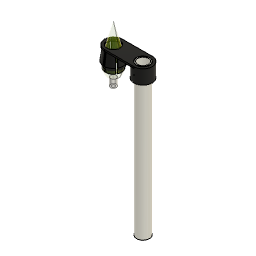
model (Autodesk Fusion 360 design; units mm, degrees)
Autodesk Fusion 360 part; units mm, degrees
note: some values were not read from the file. Chosen so that the rebuilt part matches the saved one: how an offset face is resized. Set by a fixed rule: which sketch regions a step uses.
sketch "Sketch1" plane through (0, 0, 0) normal (0, 0, 1) x (1, 0, 0)
  circle A0 centre (60, 0) radius 13.435
  circle A1 centre (0, 0) radius 13.0969
  circle A2 centre (0, 0) radius 18.0969
  circle A3 centre (60, 0) radius 18.435
  line L0 (-0.102, 18.0966) -> (59.8961, 18.4347)
  line L1 (59.8961, -18.4347) -> (-0.102, -18.0966)
  line L2 (60, 0) -> (0, 0) construction
  dimension "d4" = 26.87
  dimension "d7" = 26.1938
  dimension "d8" = 5
  dimension "d9" = 5
  dimension "d10" = 60
  constraint coincident A1.centre A2.centre
  constraint coincident A2 L0.start
  constraint coincident A3 L0.end
  constraint tangent A3 L0
  constraint tangent A2 L0
  constraint coincident A3 L1.start
  constraint coincident A2 L1.end
  constraint tangent A2 L1
  constraint tangent A3 L1
  constraint coincident A0.centre A3.centre
  constraint horizontal L2
  measures "d4" diameter of A0
  measures "d7" diameter of A1
  measures "d10" distance of A0.centre A1.centre
extrude "Extrude1" add sketch "Sketch1" against normal blind 25.4 contours A3 makes body 1
extrude "Extrude2" add sketch "Sketch1" along normal blind 3.175 bodies 1
sketch "Sketch2" plane through (0, 0, 0) normal (0, 1, 0) x (1, 0, 0)
  line L0 (13.97, 0) -> (17.4625, 25.4)
  line L1 (17.4625, 25.4) -> (13.97, 38.1)
  line L2 (0, 0) -> (0, 29) construction
  line L3 (0, 0) -> (13.97, 0) construction
  line L4 (15.9514, -0.2724) -> (19.4998, 25.5344)
  line L5 (19.4998, 25.5344) -> (15.8984, 38.6303)
  line L6 (13.97, 38.1) -> (16.0442, 38.1)
  line L7 (13.97, 0) -> (15.9888, 0)
  dimension "d15" = 13.97
  dimension "d16" = 17.4625
  dimension "d17" = 13.97
  dimension "d18" = 25.4
  dimension "d19" = 38.1
  dimension "d20" = 2
  constraint coincident L2.start L3.start
  constraint vertical L2
  constraint perpendicular L2 L3
  constraint coincident L5 L6.end
  constraint horizontal L6
  constraint coincident L4 L7.end
  constraint parallel L3 L7
  measures "d15" distance of L2.start L0.start
  measures "d16" distance of L0.end L2
  measures "d17" distance of L1.end L2
  measures "d18" distance of L0.end L3
  measures "d19" distance of L1.end L3
revolve "Revolve1" add sketch "Sketch2" angle 25 about axis through (0, 0, 1.75) along (0, 0, 1) second angle 25 bodies 1
pattern_circular "C-Pattern1" count 6 over 360 about axis through (0, 0, 1.75) along (0, 0, 1) of "Revolve1"
sketch "Sketch3" plane through (0, 0, 0) normal (0, 1, 0) x (1, 0, 0)
  line L0 (46.565, 25.4) -> (73.435, 25.4)
  line L1 (78.435, 25.4) -> (41.565, 25.4)
  line L2 (13.0969, -3.175) -> (-13.0969, -3.175)
  line L3 (73.435, -3.175) -> (46.565, -3.175)
  line L4 (-18.0969, -3.175) -> (-0.102, -3.175)
  line L5 (-0.102, -3.175) -> (59.8961, -3.175)
  line L6 (59.8961, -3.175) -> (78.435, -3.175)
  line L7 (59.8961, -3.175) -> (-0.102, -3.175)
  line L8 (60, -3.175) -> (60, 25.4) construction
  line L9 (78.435, 25.4) -> (41.565, 25.4) construction
  line L10 (41.565, 0) -> (59.8961, 0) construction
  line L11 (59.8961, 0) -> (59.8961, -3.175) construction
  line L12 (59.8961, -3.175) -> (78.435, -3.175) construction
  line L13 (59.8961, -3.175) -> (59.8961, 0) construction
  circle A0 centre (60, 11.1125) radius 0.7937
  dimension "d25" = 1.5875
  constraint coincident L3 L8.start
  constraint coincident L1 L8.end
  constraint midpoint L1 L8.end
  constraint vertical L8
  constraint midpoint L8 A0.centre
  measures "d25" diameter of A0
extrude "Extrude3" cut sketch "Sketch3" along normal through all and the other way through all bodies 1
sketch "Sketch1 (2)" plane through (0, 0, 3.175) normal (0, 0, 1) x (-1, 0, 0) in component "pipe"
  circle A0 centre (0, 0) radius 13.0969
  circle A1 centre (-60, 0) radius 13.435
  arc A2 (0.102, -18.0966) -> (0.102, 18.0966) centre (0, 0) ccw
  line L0 (0.102, 18.0966) -> (-59.8961, 18.4347)
  arc A3 (-59.8961, 18.4347) -> (-59.8961, -18.4347) centre (-60, 0) ccw
  line L1 (-59.8961, -18.4347) -> (0.102, -18.0966)
  circle A4 centre (0, 0) radius 13.335
  circle A5 centre (0, 0) radius 10.795
  dimension "d39" = 26.67
  dimension "d57" = -2.54
  constraint concentric A0 A4
  measures "d39" diameter of A4
extrude "Extrude1'" add sketch "Sketch1 (2)" against normal blind 304.8 separate body contours A0 makes body 2 in component "pipe"
sketch "Sketch1 (3)" plane through (0, 0, 0) normal (0, 1, 0) x (1, 0, 0) in component "bulb"
  spline S0 degree 5 poles (0, 0) (1.0395, 3.616) (3.0532, 10.6366) (5.8776, 20.5344) (9.2433, 32.4377) (12.7327, 45.119) (15.3994, 55.5971) (17.1378, 64.2819) (17.7502, 71.6738) (17.2267, 79.8166) (15.0803, 89.1877) (11.0925, 95.3857) (6.3138, 97.977) (2.2507, 98.552) (0, 98.552) knots 0 0 0 0 0 0 0.1 0.2 0.3 0.4 0.5 0.6 0.7 0.8 0.9 1 1 1 1 1 1
  line L0 (9.9938, 98.552) -> (-9.9938, 98.552)
  line L1 (0, 0) -> (0, 98.552)
  line L2 (17.4625, 65.7509) -> (17.4625, 78.2538)
  line L3 (0, 97.5218) -> (6, 97.5218)
  line L4 (6, 97.5218) -> (6, 113.552)
  line L5 (6, 113.552) -> (0, 113.552)
  line L6 (0, 113.552) -> (0, 97.5218)
  circle A0 centre (0, 113.552) radius 3
  line L7 (0, 113.552) -> (0, 116.552)
  point P0 (17.4625, 72.0023)
  dimension "d46" = 17.4625
  dimension "d47" = 98.552
  dimension "d49" = 6
  dimension "d50" = 15
  dimension "d52" = 6
  constraint coincident S0.start L1.start
  constraint midpoint S0.end L0
  constraint perpendicular L0 L1
  constraint vertical L1
  constraint midpoint P0 L2
  constraint vertical L2
  constraint horizontal L3
  constraint vertical L4
  constraint horizontal L5
  constraint vertical L6
  constraint coincident L1 L3.start
  constraint coincident S0 L3.end
  constraint coincident L5.end L6.start
  constraint perpendicular L5 L7
  constraint coincident A0 L7.end
  measures "d46" distance of P0 L1
  measures "d47" distance of S0.start S0.end
  measures "d49" distance of L4.end L5.end
  measures "d50" distance of S0.end L5
  measures "d52" diameter of A0
revolve "Revolve1'" add sketch "Sketch1 (3)" angle 360 about axis through (0, 0, 1.75) along (0, 0, 1) separate body contours S0 L1 L3 L6 | S0 L1 L3 | S0 L0 L4 | L0 L4 L5 L6 A0 | L5 L6 A0 | L5 A0 L7 makes body 3 in component "bulb"
thread "Thread1" "ISO Metric profile 12.0 M12x1.75 6g" major diameter 11.8335 minor diameter 9.8365 pitch 1.75 angle 60 resizes the face on face at (5.9223, -0.9625, -102.8652) on bodies 3 in component "bulb"
component "pipe" placed x (1, 0, 0) y (0, 1, 0) z (0, 0, 1) at (60, 0, 0)
component "bulb" placed x (1, 0, 0) y (0, 1, 0) z (0, 0, 1) at (0, 0, 43.552)
equation "bulbOD = 1.375 in" comment "B11-type bulb, see https://blog.1000bulbs.com/home/light-bulb-shape-guide-chandelier"
equation "height = 1.5 in"
equation "pipeOD = 1.050 in" comment "3/4\" Sch. 40"
equation "d4 = pipeOD + 2 * tol_press"
equation "tol_press = ( 0.2 mm ) / 2"
equation "tol_slide = ( 0.5 mm ) / 2"
equation "d7 = bulbOD * 0.75"
equation "d15 = ( bulbOD * 0.8 ) / 2"
equation "d16 = bulbOD / 2"
equation "d17 = ( bulbOD * 0.8 ) / 2"
equation "d18 = height * 2 / 3"
equation "d19 = height"
equation "d25 = ( 1 / 16 ) * 1 in"
equation "d39 = pipeOD"
equation "d46 = bulbOD / 2"
equation "d47 = bulbHeight"
equation "bulbHeight = 3.88 in"
equation "d49 = ( 12 / 2 ) * 1 mm"
